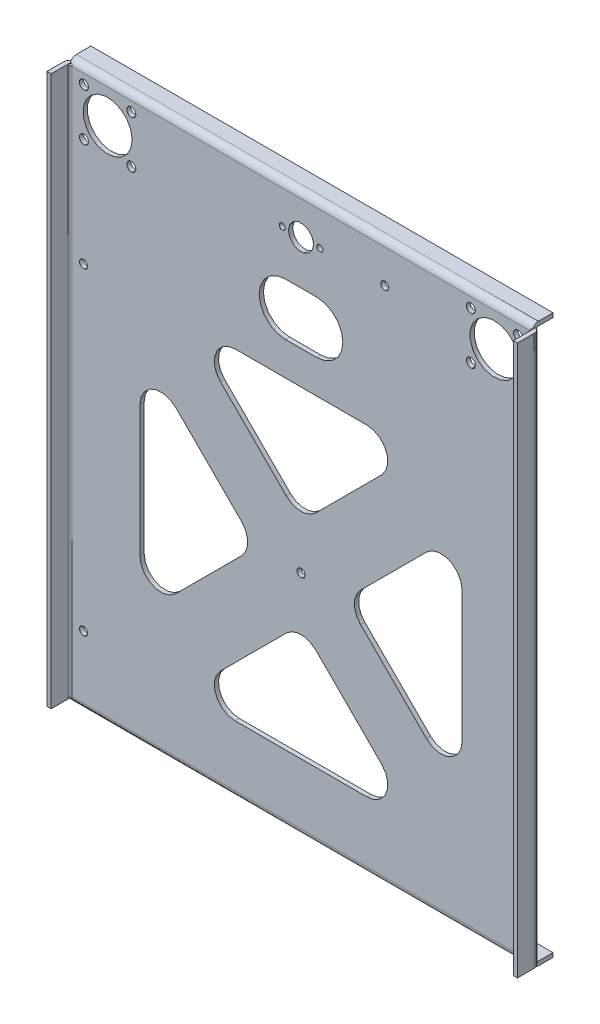
# Autodesk Inventor part: рама стола
Saved by Autodesk Inventor 2017 (Build 210142000, 142)
## iProperties
Part Number: рама стола
Material: Типовые
Document SubType Name: Modeling
Designer: Max
Mass: 108.251 g
Surface Area: 1130.64 cm^2
Volume: 108.251 cm^3
Density: 1 g/cm^3
Appearance: Резина — черная
Author: Max
Autodesk Inventor part; units mm, degrees
ref_plane "YZ Plane" through (0, 0, 0) normal (1, 0, 0) x (0, 1, 0)
ref_plane "XZ Plane" through (0, 0, 0) normal (0, 1, 0) x (-1, 0, 0)
ref_plane "XY Plane" through (0, 0, 0) normal (0, 0, 1) x (1, 0, 0)
sketch "Эскиз1" plane through (0, 0, 0) normal (0, 0, 1) x (1, 0, 0)
  circle A0 centre (0, 0.0578) radius 11.5 construction
  circle A1 centre (11.3137, -11.2559) radius 2.25 projected
  circle A2 centre (-11.3137, 11.3715) radius 2.25 projected
  circle A3 centre (-11.3137, -11.2559) radius 2.25 projected
  circle A4 centre (11.3137, 11.3715) radius 2.25 projected
  line L0 (15.5, -13.6052) -> (13.663, -15.4422) construction
  line L1 (15.5, 13.3776) -> (15.5, -13.6052) construction
  line L2 (13.3198, 15.5578) -> (15.5, 13.3776) construction
  line L3 (-13.3198, 15.5578) -> (13.3198, 15.5578) construction
  line L4 (-15.5, 13.3776) -> (-13.3198, 15.5578) construction
  line L5 (-15.5, -13.6052) -> (-15.5, 13.3776) construction
  line L6 (-13.663, -15.4422) -> (-15.5, -13.6052) construction
  line L7 (13.663, -15.4422) -> (-13.663, -15.4422) construction
  circle A5 centre (185, 0.0578) radius 11.5 construction
  circle A6 centre (196.3137, -11.2559) radius 2.25 projected
  circle A7 centre (173.6863, 11.3715) radius 2.25 projected
  circle A8 centre (173.6863, -11.2559) radius 2.25 projected
  circle A9 centre (196.3137, 11.3715) radius 2.25 projected
  line L8 (200.5, -13.6052) -> (198.663, -15.4422) construction
  line L9 (200.5, 13.3776) -> (200.5, -13.6052) construction
  line L10 (198.3198, 15.5578) -> (200.5, 13.3776) construction
  line L11 (171.6802, 15.5578) -> (198.3198, 15.5578) construction
  line L12 (169.5, 13.3776) -> (171.6802, 15.5578) construction
  line L13 (169.5, -13.6052) -> (169.5, 13.3776) construction
  line L14 (171.337, -15.4422) -> (169.5, -13.6052) construction
  line L15 (198.663, -15.4422) -> (171.337, -15.4422) construction
  circle A10 centre (101.5, 0.0578) radius 1.5 projected
  circle A11 centre (83.5, 0.0578) radius 1.5 projected
  circle A12 centre (92.5, 0.0578) radius 5 construction
  line L16 (-18, 19.0578) -> (203, 19.0578)
  line L17 (205, 17.0578) -> (205, -245.9422)
  line L18 (203, -247.9422) -> (-18, -247.9422)
  line L19 (-20, -245.9422) -> (-20, 17.0578)
  line L20 (92.5, 0.0578) -> (92.5, 19.0578) construction
  line L21 (-18, 19.0578) -> (203, 19.0578)
  line L22 (203, 17.0578) -> (-18, 17.0578)
  line L23 (-18, 17.0578) -> (-18, -245.9422)
  line L24 (-20, -245.9422) -> (-20, 17.0578)
  line L25 (203, -245.9422) -> (203, 17.0578)
  line L26 (205, 17.0578) -> (205, -245.9422)
  line L27 (-18, -247.9422) -> (203, -247.9422)
  line L28 (203, -245.9422) -> (-18, -245.9422)
  line L29 (203, -245.9422) -> (203, -247.9422)
  line L30 (203, -245.9422) -> (205, -245.9422)
  line L31 (-18, -245.9422) -> (-20, -245.9422)
  line L32 (-18, -245.9422) -> (-18, -247.9422)
  line L33 (203, 17.0578) -> (205, 17.0578)
  line L34 (203, 17.0578) -> (203, 19.0578)
  line L35 (-18, 17.0578) -> (-18, 19.0578)
  line L36 (-18, 17.0578) -> (-20, 17.0578)
  circle A13 centre (92.5, 0.0578) radius 6
  line L37 (0, 0.0578) -> (185, 0.0578) construction
  circle A14 centre (185, 0.0578) radius 11.75
  circle A15 centre (0, 0.0578) radius 11.75
  point P0 (0, 0)
  dimension "d3" = 2
  dimension "d4" = 2
  dimension "d5" = 2
  dimension "d6" = 2
  dimension "d7" = 225
  dimension "d8" = 267
  dimension "d9" = 112.5
  dimension "d10" = 112.5
  dimension "d11" = 12
  dimension "d12" = 0.0578
  dimension "d13" = 19
  dimension "d14" = 23.5
  dimension "d15" = 23.5
  constraints: 44 end point, 6 horizontal, 6 parallel, 6 perpendicular, 3 centre point, 3 coincident, 1 midpoint, 1 vertical, 1 other
  measures "d3" distance between parallel lines of L16 L22
  measures "d4" distance between parallel lines of L26 L25
  measures "d5" distance between parallel lines of L23 L24
  measures "d6" distance between parallel lines of L18 L28
  measures "d7" distance between parallel lines of L17 L19
  measures "d8" distance between parallel lines of L18 L16
  measures "d9" distance between parallel lines of L20 L24
  measures "d10" distance from line of L17 L20.start
  measures "d11" diameter of A13
  measures "d12" distance of point (0, 0) L37.start
  measures "d13" distance from line of L21 L37.start
  measures "d14" diameter of A14
  measures "d15" diameter of A15
extrude "Выдавливание1" add sketch "Эскиз1" against normal blind 2 contours L22 L25 L28 L23
extrude "Выдавливание2" add sketch "Эскиз1" against normal blind 10 contours L16 L34 L22 L35 | L28 L29 L18 L32
extrude "Выдавливание3" add sketch "Эскиз1" along normal blind 9 and the other way blind 2 contours L23 L31 L19 L36 | L33 L17 L30 L25
fillet "Сопряжение1" radius 3 4 edges at (92.5, -247.9422, 0) (92.5, 19.0578, 0) (205, -114.4422, -2) (-20, -114.4422, -2)
fillet "Сопряжение2" radius 1 4 edges at (203, -114.4422, 0) (92.5, 17.0578, -2) (92.5, -245.9422, -2) (-18, -114.4422, 0)
sketch "Эскиз2" plane through (0, 0, 0) normal (0, 0, 1) x (1, 0, 0)
  circle A0 centre (92.5, 0.0578) radius 6 projected
  line L0 (92.5, 0.0578) -> (92.5, -230.3677) construction
  circle A1 centre (92.5, -138.9422) radius 2
  line L1 (-20, 17.0578) -> (-20, -245.9422) projected
  line L2 (205, -245.9422) -> (205, 17.0578) projected
  line L3 (-18, -247.9422) -> (203, -247.9422) projected
  line L4 (15.5, -107.4422) -> (15.5, -170.4422)
  line L5 (32.5711, -177.5133) -> (64.0711, -146.0133)
  line L6 (64.0711, -131.8711) -> (32.5711, -100.3711)
  line L7 (92.5, -138.9422) -> (160.0634, -138.9422) construction
  arc A2 (64.0711, -146.0133) -> (64.0711, -131.8711) centre (57, -138.9422) ccw
  arc A3 (32.5711, -100.3711) -> (15.5, -107.4422) centre (25.5, -107.4422) ccw
  arc A4 (15.5, -170.4422) -> (32.5711, -177.5133) centre (25.5, -170.4422) ccw
  line L8 (131.0711, -198.8711) -> (99.5711, -167.3711)
  arc A5 (124, -215.9422) -> (131.0711, -198.8711) centre (124, -205.9422) ccw
  arc A6 (99.5711, -167.3711) -> (85.4289, -167.3711) centre (92.5, -174.4422) ccw
  line L9 (61, -215.9422) -> (124, -215.9422)
  arc A7 (53.9289, -198.8711) -> (61, -215.9422) centre (61, -205.9422) ccw
  line L10 (85.4289, -167.3711) -> (53.9289, -198.8711)
  line L11 (152.4289, -100.3711) -> (120.9289, -131.8711)
  arc A8 (169.5, -107.4422) -> (152.4289, -100.3711) centre (159.5, -107.4422) ccw
  arc A9 (120.9289, -131.8711) -> (120.9289, -146.0133) centre (128, -138.9422) ccw
  line L12 (169.5, -170.4422) -> (169.5, -107.4422)
  arc A10 (152.4289, -177.5133) -> (169.5, -170.4422) centre (159.5, -170.4422) ccw
  line L13 (120.9289, -146.0133) -> (152.4289, -177.5133)
  line L14 (53.9289, -79.0133) -> (85.4289, -110.5133)
  arc A11 (61, -61.9422) -> (53.9289, -79.0133) centre (61, -71.9422) ccw
  arc A12 (85.4289, -110.5133) -> (99.5711, -110.5133) centre (92.5, -103.4422) ccw
  line L15 (124, -61.9422) -> (61, -61.9422)
  arc A13 (131.0711, -79.0133) -> (124, -61.9422) centre (124, -71.9422) ccw
  line L16 (99.5711, -110.5133) -> (131.0711, -79.0133)
  line L17 (196.5, -214.9422) -> (-11.5, -214.9422) construction
  line L18 (-11.5, -214.9422) -> (-11.5, -62.9422) construction
  line L19 (-11.5, -62.9422) -> (196.5, -62.9422) construction
  line L20 (196.5, -62.9422) -> (196.5, -214.9422) construction
  line L21 (196.5, -214.9422) -> (-11.5, -62.9422) construction
  line L22 (-11.5, -214.9422) -> (196.5, -62.9422) construction
  circle A14 centre (-11.5, -62.9422) radius 2
  circle A15 centre (196.5, -62.9422) radius 2
  circle A16 centre (196.5, -214.9422) radius 2
  circle A17 centre (-11.5, -214.9422) radius 2
  line L23 (100, -33.4422) -> (85, -33.4422) construction
  line L24 (100, -20.9422) -> (85, -20.9422)
  line L25 (85, -45.9422) -> (100, -45.9422)
  arc A18 (100, -45.9422) -> (100, -20.9422) centre (100, -33.4422) ccw
  arc A19 (85, -20.9422) -> (85, -45.9422) centre (85, -33.4422) ccw
  line L26 (92.5, 0.0578) -> (132.5, 0.0578)
  circle A20 centre (132.5, 0.0578) radius 2
  point P0 (0, 0)
  point P1 (15.5, -83.3001)
  point P2 (15.5, -194.5843)
  point P3 (71.1421, -138.9422)
  point P4 (92.5, -160.3001)
  point P5 (148.1421, -215.9422)
  point P6 (36.8579, -215.9422)
  point P7 (113.8579, -138.9422)
  point P8 (169.5, -83.3001)
  point P9 (169.5, -194.5843)
  point P10 (92.5, -117.5843)
  point P11 (36.8579, -61.9422)
  point P12 (148.1421, -61.9422)
  point P13 (92.5, -33.4422)
  dimension "d26" = 4
  dimension "d27" = 112.5
  dimension "d28" = 112.5
  dimension "d29" = 109
  dimension "d33" = 10
  dimension "d34" = 10
  dimension "d35" = 87
  dimension "d36" = 51.5
  dimension "d37" = 83
  dimension "d40" = 360
  dimension "d42" = 208
  dimension "d43" = 152
  dimension "d44" = 4
  dimension "d45" = 4
  dimension "d46" = 4
  dimension "d47" = 4
  dimension "d48" = 33
  dimension "d49" = 16
  dimension "d50" = 25
  dimension "d51" = 40
  dimension "d52" = 4
  dimension "d53" = 40
  constraints: 50 end point, 28 point on circle, 27 point on line, 20 centre point, 10 tangent, 5 coincident, 3 horizontal, 3 midpoint, 3 parallel, 2 perpendicular, 2 vertical, 1 equal radius, 1 symmetric about line, 73 other
  measures "d26" diameter of A1
  measures "d27" distance from line of L1 L7.start
  measures "d28" distance from line of L2 L7.start
  measures "d29" distance from line of L3 L7.start
  measures "d33" radius of A2
  measures "d34" radius of A3
  measures "d42" distance of L18.end L19.end
  measures "d43" distance of L17.end L18.end
  measures "d44" diameter of A14
  measures "d45" diameter of A15
  measures "d46" diameter of A16
  measures "d47" diameter of A17
  measures "d48" distance between parallel lines of L3 L17
  measures "d49" distance between parallel lines of L15 L25
  measures "d50" distance between parallel lines of L25 L24
  measures "d52" diameter of A20
  measures "d53" distance of L0.start L26.end
extrude "Выдавливание4" cut sketch "Эскиз2" against normal blind 9 contours A1 | A3 L6 A2 L5 A4 L4 | A5 L9 A7 L10 A6 L8 | A8 L12 A10 L13 A9 L11 | A11 L15 A13 L16 A12 L14 | A14 | A15 | A16 | A17 | A18 L25 A19 L24 | A20
